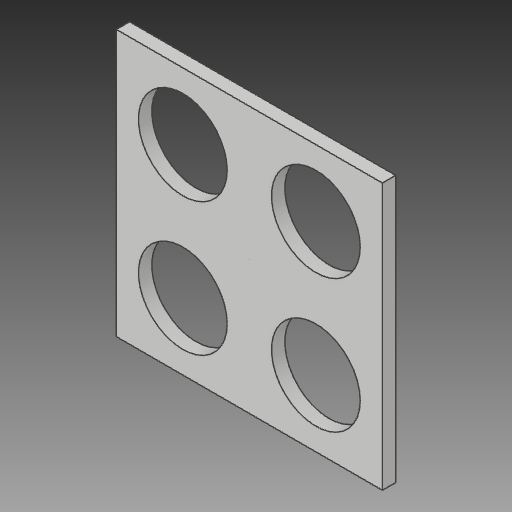
# Autodesk Inventor part: 障害物、丸４
Saved by Autodesk Inventor 2017 (Build 210142000, 142)
## iProperties
Part Number: 障害物、丸４
Material: 一般
Document SubType Name: Modeling
Designer: 雪村
Density: 1 g/cm^3
Appearance: 既定
Mass: 878.761 g
Surface Area: 1540.18 cm^2
Volume: 878.761 cm^3
Author: 雪村
Autodesk Inventor part; units mm, degrees
ref_plane "YZ Plane" through (0, 0, 0) normal (1, 0, 0) x (0, 1, 0)
ref_plane "XZ Plane" through (0, 0, 0) normal (0, 1, 0) x (-1, 0, 0)
ref_plane "XY Plane" through (0, 0, 0) normal (0, 0, 1) x (1, 0, 0)
sketch "スケッチ1" plane through (0, 0, 0) normal (0, 0, 1) x (1, 0, 0)
  line L0 (-150, 150) -> (150, 150)
  line L1 (150, 150) -> (150, -150)
  line L2 (150, -150) -> (-150, -150)
  line L3 (-150, -150) -> (-150, 150)
  circle A0 centre (-75, 75) radius 50
  circle A1 centre (-75, -75) radius 50
  circle A2 centre (75, -75) radius 50
  circle A3 centre (75, 75) radius 50
  point P0 (0, 0)
  point P1 (0, 0)
  dimension "d0" = 300
  dimension "d1" = 100
  dimension "d2" = 100
  dimension "d3" = 100
  dimension "d4" = 100
  dimension "d5" = 150
  dimension "d6" = 150
  dimension "d7" = 75
  dimension "d8" = 75
  constraints: 8 end point, 4 centre point, 2 horizontal alignment, 2 vertical alignment, 1 coincident, 1 horizontal, 9 other
  measures "d0" distance of L0.start L0.end
  measures "d1" diameter of A0
  measures "d2" diameter of A1
  measures "d3" diameter of A2
  measures "d4" diameter of A3
  measures "d5" distance of A3.centre A0.centre
  measures "d6" distance of A1.centre A0.centre
  measures "d7" distance from line of L3 A0.centre
  measures "d8" distance from line of L0 A0.centre
extrude "押し出し1" add sketch "スケッチ1" along normal blind 15
sketch "スケッチ2" plane through (0, 0, 15) normal (0, 0, 1) x (1, 0, 0)
  circle A0 centre (0, 0) radius 0.005
  dimension "d11" = 0.01
  constraints: 1 centre point, 1 coincident
  measures "d11" diameter of A0
extrude "押し出し2" cut sketch "スケッチ2" against normal through all
